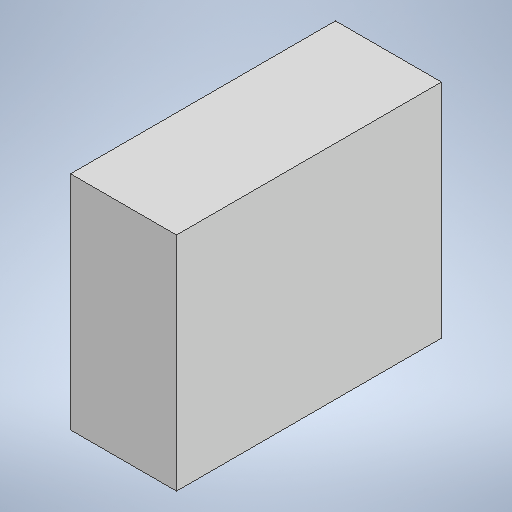
# Autodesk Inventor part: Vacuum Pump
Saved by Autodesk Inventor 2025 (Build 290162010, 162A)
## iProperties
Created: 2024-06-12
Part Number: Vacuum Pump
Material: Generic
Document SubType Name: Modeling
Designer: Alan Thomas
Mass: 17662.5 g
Surface Area: 4422 cm^2
Volume: 17662.5 cm^3
Density: 1 g/cm^3
Appearance: Default
Author: Alan Thomas
Autodesk Inventor part; units mm, degrees
ref_plane "YZ Plane" through (0, 0, 0) normal (1, 0, 0) x (0, 1, 0)
ref_plane "XZ Plane" through (0, 0, 0) normal (0, 1, 0) x (-1, 0, 0)
ref_plane "XY Plane" through (0, 0, 0) normal (0, 0, 1) x (1, 0, 0)
sketch "Sketch1" plane through (0, 0, 0) normal (0, 1, 0) x (-1, 0, 0)
  line L0 (0, -0.2486) -> (150, -0.2486)
  line L1 (150, -0.2486) -> (150, -375.2486)
  line L2 (150, -375.2486) -> (0, -375.2486)
  line L3 (0, -375.2486) -> (0, -0.2486)
  point P0 (0, 0)
  dimension "d0" = 150
  dimension "d1" = 375
  constraints: 8 end point, 2 parallel, 1 horizontal, 1 perpendicular
  measures "d0" distance of L1.end L2.end
  measures "d1" distance of L0.end L1.end
extrude "Extrusion1" add sketch "Sketch1" along normal blind 314
body "Solid1"
